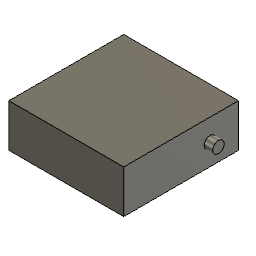
chassis (Assembly) (Autodesk Fusion 360 archive; units mm, degrees)
design "big servo demo"
part number: 2026-03-19-16-30-19-052
Autodesk Fusion 360 part; units mm, degrees
sketch "Sketch1" plane through (0, 0, 0) normal (0, 1, 0) x (1, 0, 0)
  line L0 (0, 0) -> (40, 0)
  line L1 (40, 0) -> (40, -40)
  line L2 (40, -40) -> (0, -40)
  line L3 (0, -40) -> (0, 0)
  dimension "d1" = 40
  dimension "d2" = 40
  constraint horizontal L0
  constraint vertical L1
  constraint horizontal L2
  constraint vertical L3
  constraint coincident L0.start L3.end
  measures "d1" distance of L0.start L0.end
  measures "d2" distance of L0.start L2.end
extrude "Extrude1" add sketch "Sketch1" along normal blind 15
sketch "Sketch2" plane through (40, 0, 0) normal (1, 0, 0) x (0, 0, -1)
  line L0 (-40, 0) -> (0, 0)
  line L1 (0, 0) -> (0, 15)
  line L2 (0, 15) -> (-40, 15)
  line L3 (-40, 15) -> (-40, 0)
  circle A0 centre (-10, 7.5) radius 2
  dimension "d7" = 4
  measures "d7" diameter of A0
extrude "Extrude2" add sketch "Sketch2" along normal blind 3 contours A0

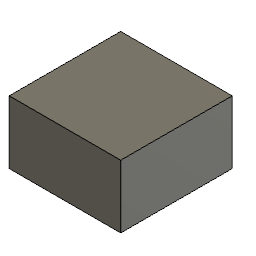
design "small servo"
part number: 2026-03-19-16-55-09-652
Autodesk Fusion 360 part; units mm, degrees
sketch "Sketch1" plane through (0, 0, 0) normal (0, 1, 0) x (1, 0, 0)
  line L0 (0, 0) -> (23, 0)
  line L1 (23, 0) -> (23, 23)
  line L2 (23, 23) -> (0, 23)
  line L3 (0, 23) -> (0, 0)
  dimension "d1" = 23
  dimension "d2" = 23
  constraint horizontal L0
  constraint vertical L1
  constraint horizontal L2
  constraint vertical L3
  constraint coincident L0.start L3.end
  measures "d1" distance of L0.start L0.end
  measures "d2" distance of L0.start L2.end
extrude "Extrude1" add sketch "Sketch1" along normal blind 13
sketch "Sketch2" plane through (0, 0, -23) normal (0, 0, -1) x (-1, 0, 0)
  line L0 (-23, 0) -> (0, 0)
  line L1 (0, 0) -> (0, 13)
  line L2 (0, 13) -> (-23, 13)
  line L3 (-23, 13) -> (-23, 0)
  circle A0 centre (-6.294, 6.5) radius 2
  dimension "d5" = 4
  measures "d5" diameter of A0
extrude "Extrude2" add sketch "Sketch2" along normal blind 3 contours A0

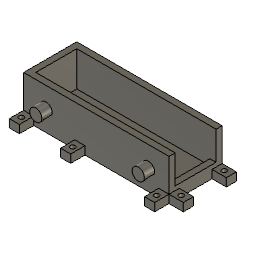
design "rezen battery holder"
Autodesk Fusion 360 part; units mm, degrees
sketch "Sketch1" plane through (0, 0, 0) normal (0, 0, 1) x (1, 0, 0)
  line L0 (-50, 70) -> (21, 70)
  line L1 (21, 70) -> (21, 44)
  line L2 (21, 44) -> (-50, 44)
  line L3 (-50, 44) -> (-50, 70)
  dimension "d1" = 71
  dimension "d2" = 26
  constraint horizontal L0
  constraint vertical L1
  constraint horizontal L2
  constraint vertical L3
  measures "d1" distance of L0.start L0.end
  measures "d2" distance of L0.start L2.end
extrude "Extrude1" add sketch "Sketch1" along normal blind 20 makes body 1
sketch "Sketch2" plane through (0, 0, 0) normal (0, 0, 1) x (1, 0, 0)
  line L0 (-50, 44) -> (21, 44)
  line L1 (21, 44) -> (21, 70)
  line L2 (21, 70) -> (-50, 70)
  line L3 (-50, 70) -> (-50, 44)
  line L4 (-50, 70) -> (-47, 70)
  line L5 (-47, 70) -> (-47, 67)
  line L6 (-47, 67) -> (-50, 67)
  line L7 (-50, 67) -> (-50, 70)
  line L8 (-50, 44) -> (-47, 44)
  line L9 (-47, 44) -> (-47, 47)
  line L10 (-47, 47) -> (-50, 47)
  line L11 (-50, 47) -> (-50, 44)
  line L12 (21, 44) -> (18, 44)
  line L13 (18, 44) -> (18, 47)
  line L14 (18, 47) -> (21, 47)
  line L15 (21, 47) -> (21, 44)
  line L16 (21, 70) -> (18, 70)
  line L17 (18, 70) -> (18, 67)
  line L18 (18, 67) -> (21, 67)
  line L19 (21, 67) -> (21, 70)
  line L20 (-47, 67) -> (18, 67)
  line L21 (18, 67) -> (18, 47)
  line L22 (18, 47) -> (-47, 47)
  line L23 (-47, 47) -> (-47, 67)
  dimension "d5" = 3
  dimension "d6" = 3
  dimension "d7" = 3
  dimension "d8" = 3
  dimension "d9" = 3
  dimension "d10" = 3
  dimension "d11" = 3
  dimension "d12" = 3
  constraint horizontal L4
  constraint vertical L5
  constraint horizontal L6
  constraint vertical L7
  constraint coincident L2.end L3.start
  constraint horizontal L8
  constraint vertical L9
  constraint horizontal L10
  constraint vertical L11
  constraint coincident L0.start L3.end
  constraint horizontal L12
  constraint vertical L13
  constraint horizontal L14
  constraint vertical L15
  constraint coincident L0.end L1.start
  constraint horizontal L16
  constraint vertical L17
  constraint horizontal L18
  constraint vertical L19
  constraint coincident L1.end L2.start
  constraint horizontal L20
  constraint vertical L21
  constraint horizontal L22
  constraint vertical L23
  measures "d5" distance of L2.end L4.end
  measures "d6" distance of L2.end L6.end
  measures "d7" distance of L0.start L8.end
  measures "d8" distance of L0.start L10.end
  measures "d9" distance of L0.end L12.end
  measures "d10" distance of L0.end L14.end
  measures "d11" distance of L1.end L16.end
  measures "d12" distance of L1.end L18.end
extrude "Extrude2" add sketch "Sketch2" along normal blind 3 separate body contours L20 L21 L22 L23 makes body 2
extrude "Extrude3" cut 1 faces at (-25.3333, 60.3333, 0) along direction (0, 0, 1) blind 25 on bodies 2 bodies 1 2
sketch "Sketch3" plane through (0, 0, 0) normal (0, 0, 1) x (1, 0, 0)
  line L0 (-47, 47) -> (18, 47)
  line L1 (18, 47) -> (18, 67)
  line L2 (18, 67) -> (-47, 67)
  line L3 (-47, 67) -> (-47, 47)
  dimension "d18" = 65
  dimension "d19" = 20
  constraint horizontal L0
  constraint vertical L1
  constraint horizontal L2
  constraint vertical L3
  measures "d18" distance of L0.start L0.end
  measures "d19" distance of L0.start L2.end
extrude "Extrude4" add sketch "Sketch3" along normal blind 3 bodies 1 2
sketch "Sketch4" plane through (0, 44, 0) normal (0, -1, 0) x (1, 0, 0)
  line L0 (-50, 0) -> (21, 0)
  line L1 (21, 0) -> (21, 20)
  line L2 (21, 20) -> (-50, 20)
  line L3 (-50, 20) -> (-50, 0)
  line L4 (-50, 0) -> (-45, 0)
  line L5 (-45, 0) -> (-45, 4)
  line L6 (-45, 4) -> (-50, 4)
  line L7 (-50, 4) -> (-50, 0)
  line L8 (-25, 0) -> (-20, 0)
  line L9 (-20, 0) -> (-20, 4)
  line L10 (-20, 4) -> (-25, 4)
  line L11 (-25, 4) -> (-25, 0)
  line L12 (16, 0) -> (21, 0)
  line L13 (21, 0) -> (21, 4)
  line L14 (21, 4) -> (16, 4)
  line L15 (16, 4) -> (16, 0)
  constraint horizontal L4
  constraint vertical L5
  constraint horizontal L6
  constraint vertical L7
  constraint coincident L0.start L3.end
  constraint horizontal L8
  constraint vertical L9
  constraint horizontal L10
  constraint vertical L11
  constraint coincident L0 L8.start
  constraint horizontal L12
  constraint vertical L13
  constraint horizontal L14
  constraint vertical L15
  constraint coincident L1 L13.end
  constraint coincident L0 L12.start
extrude "Extrude5" add sketch "Sketch4" along normal blind 7 contours L0 L3 L4 L5 L6 L7 | L0 L8 L9 L10 L11 | L0 L1 L12 L13 L14 L15 bodies 1
move_body "Move1" bodies 1 to x (1, 0, 0) y (0, 1, 0) z (0, 0, 1) at (-21, -30, 0)
sketch "Sketch5" plane through (0, 0, 0) normal (1, 0, 0) x (0, 1, 0)
  line L0 (7, 0) -> (40, 0)
  line L1 (40, 0) -> (40, 20)
  line L2 (40, 20) -> (14, 20)
  line L3 (14, 20) -> (14, 4)
  line L4 (14, 4) -> (7, 4)
  line L5 (7, 4) -> (7, 0)
  line L6 (14, 4) -> (19, 4)
  line L7 (19, 4) -> (19, 0)
  line L8 (19, 0) -> (14, 0)
  line L9 (14, 0) -> (14, 4)
  line L10 (40, 0) -> (35, 0)
  line L11 (35, 0) -> (35, 4)
  line L12 (35, 4) -> (40, 4)
  line L13 (40, 4) -> (40, 0)
  dimension "d24" = 5
  dimension "d25" = 5
  dimension "d26" = 4
  constraint horizontal L6
  constraint vertical L7
  constraint horizontal L8
  constraint vertical L9
  constraint coincident L3.end L4.start
  constraint horizontal L10
  constraint vertical L11
  constraint horizontal L12
  constraint vertical L13
  constraint coincident L0.end L1.start
  measures "d24" distance of L3.end L6.end
  measures "d25" distance of L0.end L10.end
  measures "d26" distance of L0.end L12.end
extrude "Extrude6" add sketch "Sketch5" along normal blind 7 contours L0 L6 L7 L8 L9 | L0 L1 L10 L11 L12 L13 bodies 1
sketch "Sketch6" plane through (0, 0, 0) normal (0, 0, 1) x (1, 0, 0)
  line L0 (-66, 14) -> (-71, 14)
  line L1 (-71, 14) -> (-71, 7)
  line L2 (-71, 7) -> (-66, 7)
  line L3 (-66, 7) -> (-66, 14)
  line L4 (-41, 14) -> (-46, 14)
  line L5 (-46, 14) -> (-46, 7)
  line L6 (-46, 7) -> (-41, 7)
  line L7 (-41, 7) -> (-41, 14)
  line L8 (0, 14) -> (-5, 14)
  line L9 (-5, 14) -> (-5, 7)
  line L10 (-5, 7) -> (0, 7)
  line L11 (0, 7) -> (0, 14)
  line L12 (0, 14) -> (7, 14)
  line L13 (0, 19) -> (0, 14)
  line L14 (0, 14) -> (7, 14)
  line L15 (7, 14) -> (7, 19)
  line L16 (7, 19) -> (0, 19)
  line L17 (0, 40) -> (0, 35)
  line L18 (0, 35) -> (7, 35)
  line L19 (7, 35) -> (7, 40)
  line L20 (7, 40) -> (0, 40)
  line L21 (-68, 17) -> (-68, 37)
  line L22 (-68, 37) -> (-3, 37)
  line L23 (-3, 37) -> (-3, 17)
  line L24 (-3, 17) -> (-68, 17)
  line L25 (-71, 14) -> (0, 14)
  line L26 (0, 14) -> (0, 40)
  line L27 (0, 40) -> (-71, 40)
  line L28 (-71, 40) -> (-71, 14)
  line L29 (-66, 14) -> (-66, 10.5)
  line L30 (-66, 10.5) -> (-68.5, 10.5)
  line L31 (-41, 14) -> (-41, 10.5)
  line L32 (-41, 10.5) -> (-43.5, 10.5)
  line L33 (0, 14) -> (0, 10.5)
  line L34 (0, 10.5) -> (-2.5, 10.5)
  line L35 (0, 14) -> (3.5, 14)
  line L36 (3.5, 14) -> (3.5, 16.5)
  line L37 (0, 35) -> (3.5, 35)
  line L38 (3.5, 35) -> (3.5, 37.5)
  circle A0 centre (3.5, 37.5) radius 1.2
  circle A1 centre (3.5, 16.5) radius 1.2
  circle A2 centre (-2.5, 10.5) radius 1.2
  circle A3 centre (-43.5, 10.5) radius 1.2
  circle A4 centre (-68.5, 10.5) radius 1.2
  dimension "d29" = 3.5
  dimension "d30" = 2.5
  dimension "d31" = 3.5
  dimension "d32" = 2.5
  dimension "d33" = 2.5
  dimension "d34" = 2.5
  dimension "d35" = 2.4
  dimension "d36" = 2.4
  dimension "d37" = 2.4
  dimension "d38" = 2.4
  dimension "d39" = 2.4
  constraint coincident L0.start L3.end
  constraint perpendicular L25 L29
  constraint perpendicular L3 L30
  constraint coincident L4.start L7.end
  constraint perpendicular L25 L31
  constraint perpendicular L7 L32
  constraint coincident L8.start L11.end
  constraint midpoint L11 L33.end
  constraint perpendicular L33 L34
  constraint midpoint L12 L35.end
  constraint perpendicular L14 L36
  constraint coincident L17.end L18.start
  constraint midpoint L18 L37.end
  constraint perpendicular L18 L38
  constraint coincident L38.end A0.centre
  constraint coincident L36.end A1.centre
  constraint coincident L34.end A2.centre
  constraint coincident L32.end A3.centre
  constraint coincident L30.end A4.centre
  measures "d29" distance of L0.start L29.end
  measures "d30" distance of L29.end L30.end
  measures "d31" distance of L4.start L31.end
  measures "d32" distance of L31.end L32.end
  measures "d33" distance of L33.end L34.end
  measures "d34" distance of L35.end L36.end
  measures "d35" diameter of A0
  measures "d36" diameter of A1
  measures "d37" diameter of A2
  measures "d38" diameter of A3
  measures "d39" diameter of A4
extrude "Extrude7" cut sketch "Sketch6" along normal blind 5 contours A0 | A1 | A2 | A3 | A4 bodies 1
sketch "Sketch7" plane through (0, 14, 0) normal (0, -1, 0) x (1, 0, 0)
  line L0 (-5, 0) -> (-5, 4)
  line L1 (-5, 4) -> (0, 4)
  line L2 (0, 4) -> (0, 20)
  line L3 (0, 20) -> (-71, 20)
  line L4 (-71, 20) -> (-71, 4)
  line L5 (-71, 4) -> (-66, 4)
  line L6 (-66, 4) -> (-66, 0)
  line L7 (-66, 0) -> (-46, 0)
  line L8 (-46, 0) -> (-46, 4)
  line L9 (-46, 4) -> (-41, 4)
  line L10 (-41, 4) -> (-41, 0)
  line L11 (-41, 0) -> (-5, 0)
  line L12 (-60, 10) -> (-10, 10)
  circle A0 centre (-60, 10) radius 3
  circle A1 centre (-10, 10) radius 3
  dimension "d42" = 6
  dimension "d43" = 6
  constraint horizontal L12
  constraint coincident L12.start A0.centre
  constraint coincident L12.end A1.centre
  measures "d42" diameter of A0
  measures "d43" diameter of A1
extrude "Extrude8" add sketch "Sketch7" along normal blind 5 contours A0 | A1 bodies 1
sketch "Sketch8" plane through (0, 40, 0) normal (0, 1, 0) x (-1, 0, 0)
  line L0 (-7, 0) -> (71, 0)
  line L1 (71, 0) -> (71, 20)
  line L2 (71, 20) -> (0, 20)
  line L3 (0, 20) -> (0, 4)
  line L4 (0, 4) -> (-7, 4)
  line L5 (-7, 4) -> (-7, 0)
  line L6 (60, 10) -> (10, 10)
  line L7 (10, 10) -> (10, 20)
  line L8 (10, 20) -> (10, 10)
  circle A0 centre (10, 10) radius 3
  circle A1 centre (60, 10) radius 3
  dimension "d46" = 6
  dimension "d47" = 6
  constraint horizontal L6
  constraint coincident L2 L7.end
  constraint perpendicular L2 L7
  constraint coincident L6.end L7.start
  constraint coincident L6.start A1.centre
  measures "d46" diameter of A0
  measures "d47" diameter of A1
extrude "Extrude9" add sketch "Sketch8" along normal blind 5 contours L6 L7 L8 A0 | L6 L7 L8 A0 | A1 bodies 1
sketch "Sketch9" plane through (0, 0, 0) normal (1, 0, 0) x (0, 1, 0)
  line L0 (35, 0) -> (35, 4)
  line L1 (35, 4) -> (40, 4)
  line L2 (40, 4) -> (40, 20)
  line L3 (40, 20) -> (14, 20)
  line L4 (14, 20) -> (14, 4)
  line L5 (14, 4) -> (19, 4)
  line L6 (19, 4) -> (19, 0)
  line L7 (19, 0) -> (35, 0)
  line L8 (10, 9) -> (14, 9)
  line L9 (14, 9) -> (14, 7)
  line L10 (14, 7) -> (10, 7)
  line L11 (10, 7) -> (10, 9)
  line L12 (44, 9) -> (40, 9)
  line L13 (40, 9) -> (40, 7)
  line L14 (40, 7) -> (44, 7)
  line L15 (44, 7) -> (44, 9)
  constraint horizontal L8
  constraint vertical L9
  constraint horizontal L10
  constraint vertical L11
  constraint coincident L4 L9.end
  constraint horizontal L12
  constraint vertical L13
  constraint horizontal L14
  constraint vertical L15
  constraint coincident L2 L13.end
extrude "Extrude10" cut sketch "Sketch9" against normal blind 70 contours L2 L12 L13 L14 L15 | L4 L8 L9 L10 L11 bodies 1
sketch "Sketch10" plane through (0, 0, 20) normal (0, 0, 1) x (-1, 0, 0)
  line L0 (68, -17) -> (68, -37)
  line L1 (68, -37) -> (3, -37)
  line L2 (3, -37) -> (3, -17)
  line L3 (3, -17) -> (68, -17)
  line L4 (71, -14) -> (0, -14)
  line L5 (0, -14) -> (0, -40)
  line L6 (0, -40) -> (71, -40)
  line L7 (71, -40) -> (71, -14)
  line L8 (3, -17) -> (0, -17)
  line L9 (0, -17) -> (0, -37)
  line L10 (0, -37) -> (3, -37)
  line L11 (3, -37) -> (3, -17)
  dimension "d54" = 3
  dimension "d55" = 20
  constraint horizontal L8
  constraint vertical L9
  constraint horizontal L10
  constraint vertical L11
  constraint coincident L2.end L3.start
  measures "d54" distance of L2.end L8.end
  measures "d55" distance of L2.end L1.end
extrude "Extrude11" cut sketch "Sketch10" against normal blind 14 contours L2 L5 L8 L9 L10 L11 bodies 1

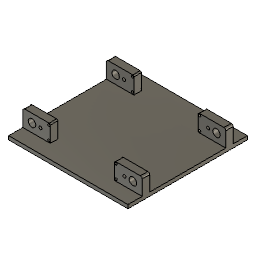
design "chassis"
Autodesk Fusion 360 part; units mm, degrees
sketch "Sketch2" plane through (0, 0, 0) normal (0, 0, 1) x (1, 0, 0)
  line L0 (-40, 40) -> (40, 40)
  line L1 (40, 40) -> (40, 0)
  line L2 (40, 0) -> (-40, 0)
  line L3 (-40, 0) -> (-40, 40)
  constraint horizontal L0
  constraint vertical L1
  constraint horizontal L2
  constraint vertical L3
extrude "Extrude2" add sketch "Sketch2" along normal blind 5 makes body 1
sketch "Sketch3" plane through (0, 0, 5) normal (0, 0, 1) x (-1, 0, 0)
  line L0 (40, 0) -> (-40, 0)
  line L1 (-40, 0) -> (-40, -40)
  line L2 (-40, -40) -> (40, -40)
  line L3 (40, -40) -> (40, 0)
  line L4 (40.4995, -21.0066) -> (3.0495, -21.0012)
  line L5 (3.0495, -21.0012) -> (3.0509, -11.0012)
  line L6 (3.0509, -11.0012) -> (40, -11.0012)
  dimension "d11" = 19
  dimension "d12" = 37.45
  dimension "d13" = 10
  constraint perpendicular L4 L5
  constraint coincident L3 L6.end
  constraint perpendicular L3 L6
  measures "d11" distance of L2.end L4.start
  measures "d12" distance of L4.start L4.end
  measures "d13" distance of L4.end L5.end
extrude "Extrude3" add sketch "Sketch3" along normal blind 22.65 contours L3 L4 L5 L6 bodies 1
sketch "Sketch4" plane through (0, 0, 0) normal (0, 1, 0) x (1, 0, 0)
  line L0 (-3.0495, -5) -> (-40, -5)
  line L1 (-40, -5) -> (-40, -27.65)
  line L2 (-40, -27.65) -> (-3.0495, -27.65)
  line L3 (-3.0495, -27.65) -> (-3.0495, -5)
  circle A0 centre (-4.9995, -25.125) radius 1.5
  circle A1 centre (-4.9995, -7.525) radius 1.5
  circle A2 centre (-16.2995, -16.325) radius 2
  circle A3 centre (-27.5495, -16.325) radius 5
  dimension "d19" = 3
  dimension "d22" = 3
  dimension "d25" = 4
  dimension "d26" = 11.25
  dimension "d27" = 10
  measures "d19" diameter of A0
  measures "d22" diameter of A1
  measures "d25" diameter of A2
  measures "d26" distance of A2.centre A3.centre
  measures "d27" diameter of A3
sketch "Sketch6" plane through (0, 0, 0) normal (0, 1, 0) x (1, 0, 0)
extrude "Extrude5" cut sketch "Sketch4" along normal blind 25 contours A0 | A1 | A2 | A3 bodies 1
fillet "Fillet3" radius 1.5 1 edges at (-3.0502, 16.0012, 27.65) on bodies 1
fillet "Fillet4" radius 2.5 1 edges at (-40, 16.0038, 27.65) on bodies 1
move_body "Move1" bodies 1 to x (1, 0, 0) y (0, 1, 0) z (0, 0, 1) at (-40, 0, 0)
move_body "Move2" bodies 1 to x (1, 0, 0) y (0, 1, 0) z (0, 0, 1) at (0, 40, 0)
mirror "Mirror1" about plane through (0, 0, 0) normal (1, 0, 0) of bodies 1 merged
mirror "Mirror2" about plane through (0, 0, 0) normal (0, 1, 0) of bodies 1 makes body 2
sketch "Sketch7" plane through (0, 0, 0) normal (0, 0, 1) x (1, 0, 0)
extrude "Extrude6" add 1 faces at (26.6667, 40, 1.6667) along direction (0, -1, 0) blind 80 on bodies 1 bodies 1 2

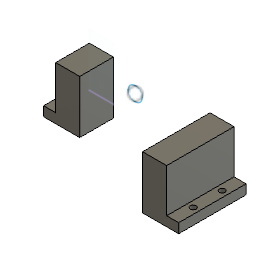
design "servo holder"
part number: 2026-03-16-18-08-13-448
Autodesk Fusion 360 part; units mm, degrees
sketch "Sketch2" plane through (0, 5, 0) normal (0, 1, 0) x (-1, 0, 0)
  line L0 (-160, 0) -> (0, 0)
  line L1 (0, 0) -> (0, 160)
  line L2 (0, 160) -> (-160, 160)
  line L3 (-160, 160) -> (-160, 0)
  line L4 (-160, 80) -> (0, 80)
  line L5 (0, 80) -> (-160, 80)
  line L6 (-160, 80) -> (-160, 92)
  line L7 (-160, 92) -> (0, 92)
  line L8 (0, 92) -> (0, 80)
  line L9 (0, 92) -> (-60, 92)
  line L10 (-60, 92) -> (-60, 120)
  line L11 (-60, 120) -> (0, 120)
  line L12 (0, 120) -> (0, 92)
  line L13 (-160, 92) -> (-100, 92)
  line L14 (-100, 92) -> (-100, 120)
  line L15 (-100, 120) -> (-160, 120)
  line L16 (-160, 120) -> (-160, 92)
  line L17 (-60, 92) -> (-50, 92)
  line L18 (-50, 92) -> (-50, 120)
  line L19 (-50, 120) -> (-60, 120)
  line L20 (-60, 120) -> (-60, 92)
  line L21 (-100, 92) -> (-110, 92)
  line L22 (-110, 92) -> (-110, 120)
  line L23 (-110, 120) -> (-100, 120)
  line L24 (-100, 120) -> (-100, 92)
  dimension "d7" = 160
  dimension "d8" = 12
  dimension "d9" = 60
  dimension "d10" = 28
  dimension "d11" = 60
  dimension "d12" = 28
  dimension "d13" = 10
  dimension "d14" = 28
  dimension "d15" = 10
  dimension "d16" = 28
  constraint midpoint L3 L4.start
  constraint midpoint L1 L4.end
  constraint horizontal L5
  constraint vertical L6
  constraint horizontal L7
  constraint vertical L8
  constraint horizontal L9
  constraint vertical L10
  constraint horizontal L11
  constraint vertical L12
  constraint horizontal L13
  constraint vertical L14
  constraint horizontal L15
  constraint vertical L16
  constraint horizontal L17
  constraint vertical L18
  constraint horizontal L19
  constraint vertical L20
  constraint horizontal L21
  constraint vertical L22
  constraint horizontal L23
  constraint vertical L24
  measures "d7" distance of L4.end L4.start
  measures "d8" distance of L4.end L7.end
  measures "d9" distance of L7.end L9.end
  measures "d10" distance of L7.end L11.end
  measures "d11" distance of L6.end L13.end
  measures "d12" distance of L6.end L15.end
  measures "d13" distance of L9.end L17.end
  measures "d14" distance of L9.end L10.end
  measures "d15" distance of L13.end L21.end
  measures "d16" distance of L13.end L14.end
extrude "Extrude2" add sketch "Sketch2" along normal blind 22 contours L7 L13 L14 L15 L21 L22 L23 L24 | L7 L9 L10 L11 L17 L18 L19 L20 makes body 1 at (60, 12.3333, 101.3333) makes body 2 at (110, 12.3333, 101.3333)
sketch "Sketch3" plane through (0, 0, 92) normal (0, 0, -1) x (-1, 0, 0)
  line L0 (-100, 5) -> (-100, 27)
  line L1 (-100, 27) -> (-110, 27)
  line L2 (-110, 27) -> (-110, 5)
  line L3 (-105, 5) -> (-105, 7.3)
  circle A0 centre (-105, 9.45) radius 2.15
  circle A1 centre (-105.1004, 19.2477) radius 2.15
  line L4 (-105, 9.45) -> (-105.1004, 19.2477)
  line L5 (-55, 5) -> (-55, 7.3)
  circle A2 centre (-55, 9.45) radius 2.15
  line L6 (-55, 9.45) -> (-55, 19.248)
  circle A3 centre (-55, 19.248) radius 2.15
  circle A4 centre (-105.1004, 19.2477) radius 0.9
  circle A5 centre (-105, 9.45) radius 0.9
  circle A6 centre (-55, 9.45) radius 0.9
  circle A7 centre (-55, 19.248) radius 0.9
  line L7 (-110, 5) -> (-100, 5)
  dimension "d19" = 2.3
  dimension "d20" = 2.15
  dimension "d23" = 2.3
  dimension "d24" = 2.15
  dimension "d26" = 9.798
  dimension "d27" = 4.3
  dimension "d28" = 1.8
  dimension "d29" = 1.8
  dimension "d30" = 1.8
  dimension "d31" = 1.8
  constraint coincident L3.end A0
  constraint coincident A0.centre L4.start
  constraint coincident A1.centre L4.end
  constraint vertical L5
  constraint coincident L5.end A2
  constraint coincident A2.centre L6.start
  constraint vertical L6
  constraint coincident L6.end A3.centre
  constraint concentric A1 A4
  constraint concentric A0 A5
  constraint concentric A2 A6
  constraint concentric A3 A7
  measures "d19" distance of L3.start L3.end
  measures "d20" distance of L3.end A0.centre
  measures "d23" distance of L5.start L5.end
  measures "d24" distance of L5.end A2.centre
  measures "d26" distance of A2.centre L6.end
  measures "d27" diameter of A3
  measures "d28" diameter of A4
  measures "d29" diameter of A5
  measures "d30" diameter of A6
  measures "d31" diameter of A7
extrude "Extrude3" cut sketch "Sketch3" against normal blind 10 contours A4 | A5 | A6 | A7 bodies 1 2
sketch "Sketch4" plane through (0, 0, 92) normal (0, 0, -1) x (-1, 0, 0)
  circle A0 centre (-55, 9.45) radius 0.9
  circle A1 centre (-55, 19.248) radius 0.9
  line L0 (-50, 5) -> (-50, 27)
  line L1 (-50, 27) -> (-60, 27)
  line L2 (-60, 27) -> (-60, 5)
  line L3 (-60, 5) -> (-50, 5)
  circle A2 centre (-69, 13.3) radius 2.9
  dimension "d37" = 5.8
  measures "d37" diameter of A2
sketch "Sketch5" plane through (0, 0, 0) normal (0, 1, 0) x (1, 0, 0)
  line L0 (60, -120) -> (60, -92)
  line L1 (60, -92) -> (50, -92)
  line L2 (50, -92) -> (50, -120)
  line L3 (50, -120) -> (60, -120)
  line L4 (100, -120) -> (110, -120)
  line L5 (110, -120) -> (110, -92)
  line L6 (110, -92) -> (100, -92)
  line L7 (100, -92) -> (100, -120)
  line L8 (95, -92) -> (100, -92)
  line L9 (100, -92) -> (100, -120)
  line L10 (110, -120) -> (115, -120)
  line L11 (115, -120) -> (115, -92)
  line L12 (115, -92) -> (110, -92)
  line L13 (110, -92) -> (110, -120)
  line L14 (100, -120) -> (95, -120)
  line L15 (95, -120) -> (95, -92)
  line L16 (95, -92) -> (100, -92)
  line L17 (100, -92) -> (100, -120)
  line L18 (60, -120) -> (65, -120)
  line L19 (65, -120) -> (65, -92)
  line L20 (65, -92) -> (60, -92)
  line L21 (60, -92) -> (60, -120)
  line L22 (50, -120) -> (45, -120)
  line L23 (45, -120) -> (45, -92)
  line L24 (45, -92) -> (50, -92)
  line L25 (50, -92) -> (50, -120)
  dimension "d40" = 28
  dimension "d41" = 5
  dimension "d42" = 28
  dimension "d43" = 5
  dimension "d44" = 5
  dimension "d45" = 28
  dimension "d46" = 5
  dimension "d47" = 28
  constraint horizontal L8
  constraint vertical L9
  constraint coincident L4.start L7.end
  constraint horizontal L10
  constraint vertical L11
  constraint horizontal L12
  constraint vertical L13
  constraint coincident L4.end L5.start
  constraint horizontal L14
  constraint vertical L15
  constraint horizontal L16
  constraint vertical L17
  constraint horizontal L18
  constraint vertical L19
  constraint horizontal L20
  constraint vertical L21
  constraint coincident L0.start L3.end
  constraint horizontal L22
  constraint vertical L23
  constraint horizontal L24
  constraint vertical L25
  constraint coincident L2.end L3.start
  measures "d40" distance of L4.start L6.end
  measures "d41" distance of L4.end L10.end
  measures "d42" distance of L4.end L5.end
  measures "d43" distance of L4.start L14.end
  measures "d44" distance of L0.start L18.end
  measures "d45" distance of L0.start L0.end
  measures "d46" distance of L2.end L22.end
  measures "d47" distance of L2.end L1.end
move_body "Move1" bodies 1 2 to x (1, 0, 0) y (0, 1, 0) z (0, 0, 1) at (0, -5, 0)
extrude "Extrude5" add sketch "Sketch5" along normal blind 4 contours L0 L18 L19 L20 L21 | L2 L22 L23 L24 L25 | L7 L8 L9 L14 L15 L16 L17 | L5 L10 L11 L12 L13 bodies 1 2
sketch "Sketch6" plane through (0, 4, 0) normal (0, 1, 0) x (-1, 0, 0)
  line L0 (-100, 92) -> (-95, 92)
  line L1 (-95, 92) -> (-95, 120)
  line L2 (-95, 120) -> (-100, 120)
  line L3 (-100, 120) -> (-100, 92)
  circle A0 centre (-97.5136, 111.5) radius 1.2
  circle A1 centre (-97.5136, 99.5) radius 1.2
  circle A2 centre (-112.5136, 111.5) radius 1.2
  circle A3 centre (-112.5136, 99.5) radius 1.2
  circle A4 centre (-47.5136, 111.5) radius 1.2
  circle A5 centre (-62.5136, 111.5) radius 1.2
  circle A6 centre (-62.5136, 99.5) radius 1.2
  circle A7 centre (-47.5136, 99.5) radius 1.2
  dimension "d54" = 2.4
  dimension "d55" = 2.4
  dimension "d56" = 2.4
  dimension "d57" = 2.4
  dimension "d58" = 2.4
  dimension "d59" = 2.4
  dimension "d60" = 2.4
  dimension "d61" = 2.4
  measures "d54" diameter of A0
  measures "d55" diameter of A1
  measures "d56" diameter of A2
  measures "d57" diameter of A3
  measures "d58" diameter of A4
  measures "d59" diameter of A7
  measures "d60" diameter of A5
  measures "d61" diameter of A6
extrude "Extrude6" cut sketch "Sketch6" against normal blind 10 contours A0 | A1 | A2 | A3 | A4 | A5 | A6 | A7 bodies 1 2
sketch "Sketch7" plane through (0, 0, 92) normal (0, 0, -1) x (-1, 0, 0)
  circle A0 centre (-105, 4.45) radius 0.9
  circle A1 centre (-105.1004, 14.2477) radius 0.9
  line L0 (-115, 0) -> (-95, 0)
  line L1 (-95, 0) -> (-95, 4)
  line L2 (-95, 4) -> (-100, 4)
  line L3 (-100, 4) -> (-100, 22)
  line L4 (-100, 22) -> (-110, 22)
  line L5 (-110, 22) -> (-110, 4)
  line L6 (-110, 4) -> (-115, 4)
  line L7 (-115, 4) -> (-115, 0)
  line L8 (-100, 4) -> (-60, 4)
  line L9 (-60, 4) -> (-60, 0)
  line L10 (-60, 0) -> (-100, 0)
  line L11 (-100, 0) -> (-100, 4)
  constraint horizontal L8
  constraint vertical L9
  constraint horizontal L10
  constraint vertical L11
  constraint coincident L2.end L3.start
extrude "Extrude7" cut sketch "Sketch7" against normal blind 100 contours L0 L1 L2 L8 L10 L11 | L1 L8 L9 L10 bodies 1 2
sketch "Sketch8" plane through (50, 0, 0) normal (-1, 0, 0) x (0, 0, 1)
  line L0 (92, 4) -> (120, 4)
  line L1 (120, 4) -> (120, 22)
  line L2 (120, 22) -> (92, 22)
  line L3 (92, 22) -> (92, 4)
  line L4 (92, 0) -> (106, 0)
  line L5 (106, 0) -> (106, 22)
  line L6 (106, 22) -> (92, 22)
  line L7 (92, 22) -> (92, 0)
  line L8 (106, 22) -> (120, 22)
  line L9 (120, 22) -> (120, 0)
  line L10 (120, 0) -> (106, 0)
  line L11 (106, 0) -> (106, 22)
  dimension "d66" = 14
  dimension "d67" = 22
  constraint horizontal L4
  constraint vertical L5
  constraint horizontal L6
  constraint vertical L7
  constraint horizontal L8
  constraint vertical L9
  constraint horizontal L10
  constraint vertical L11
  measures "d66" distance of L4.start L4.end
  measures "d67" distance of L4.start L2.end
extrude "Extrude8" cut sketch "Sketch8" along normal blind 17 and the other way blind 32 contours L0 L1 L2 L5 L8 L9 L11 | L0 L5 L9 L10 L11 bodies 1
